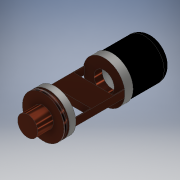
# Autodesk Inventor part: Part 3 of Focusrite Microphone
Saved by Autodesk Inventor 2018 (Build 220112000, 112)
## iProperties
Created: 2017-11-13
Part Number: Part 3 of Focusrite Microphone
Material: Generic
Document SubType Name: Modeling
Designer: Justin
Density: 1 g/cm^3
Appearance: Default
Author: Justin
Autodesk Inventor part; units mm, degrees
ref_plane "YZ Plane" through (0, 0, 0) normal (1, 0, 0) x (0, 1, 0)
ref_plane "XZ Plane" through (0, 0, 0) normal (0, 1, 0) x (-1, 0, 0)
ref_plane "XY Plane" through (0, 0, 0) normal (0, 0, 1) x (1, 0, 0)
sketch "Sketch1" plane through (0, 0, 0) normal (0, 0, 1) x (1, 0, 0)
  line L0 (0, 0) -> (12.3503, 0)
  line L1 (12.3503, 0) -> (12.3503, 19)
  line L2 (12.3503, 19) -> (0, 19)
  line L3 (0, 19) -> (0, 0)
  line L4 (0, 19) -> (25.485, 19)
  line L5 (25.485, 19) -> (25.485, 22.5)
  line L6 (25.485, 22.5) -> (0, 22.5)
  line L7 (0, 22.5) -> (0, 19)
  line L8 (23.226, 22.5) -> (23.226, 25.5)
  line L9 (23.226, 25.5) -> (0, 25.5)
  line L10 (0, 25.5) -> (0, 22.5)
  line L11 (23.226, 25.5) -> (25.485, 25.5)
  line L12 (25.485, 25.5) -> (25.485, 33.5)
  line L13 (25.485, 33.5) -> (20.485, 33.5)
  line L14 (20.485, 33.5) -> (20.485, 22.5)
  dimension "d0" = 19
  dimension "d1" = 25.485
  dimension "d2" = 3.5
  dimension "d3" = 90
  dimension "d4" = 3
  dimension "d5" = 8
  dimension "d6" = 5
  constraints: 30 end point, 11 perpendicular, 5 point on line, 1 horizontal, 1 parallel
  measures "d0" distance of L0.end L1.end
  measures "d1" distance of L2.end L4.end
  measures "d2" distance of L4.end L5.end
  measures "d3" angle of L5 L4
  measures "d4" distance of L8.start L8.end
  measures "d5" distance of L11.end L12.end
  measures "d6" distance of L12.end L13.end
revolve "Revolution1" add sketch "Sketch1" angle 360 about axis through (0, 19, 0) along (0, -1, 0)
sketch "Sketch2" plane through (0, 33.5, 0) normal (0, 1, 0) x (1, 0, 0)
  line L0 (25.0712, -4.4185) -> (24.0712, -4.4185)
  line L1 (24.0712, -4.4185) -> (24.0712, 4.5815)
  line L2 (24.0712, 4.5815) -> (25.0712, 4.5815)
  line L3 (25.0712, 4.5815) -> (25.0712, -4.4185)
  line L4 (-23.9768, -4.4185) -> (-24.9768, -4.4185)
  line L5 (-24.9768, -4.4185) -> (-24.9768, 4.5815)
  line L6 (-24.9768, 4.5815) -> (-23.9768, 4.5815)
  line L7 (-23.9768, 4.5815) -> (-23.9768, -4.4185)
  point P0 (0, 0)
  dimension "d8" = 1
  dimension "d9" = 9
  dimension "d10" = 1
  dimension "d11" = 9
  constraints: 16 end point, 4 parallel, 2 horizontal, 2 perpendicular, 1 point on line
  measures "d8" distance of L1.end L2.end
  measures "d9" distance of L0.end L1.end
  measures "d10" distance of L5.end L6.end
  measures "d11" distance of L4.end L5.end
extrude "Extrusion1" add sketch "Sketch2" along normal blind 60
sketch "Sketch3" plane through (0, 93.5, 0) normal (0, 1, 0) x (1, 0, 0)
  circle A0 centre (0, 0) radius 12.3503 projected
  circle A1 centre (0, 0) radius 25.485
  constraints: 1 centre point, 1 coincident
extrude "Extrusion2" add sketch "Sketch3" along normal blind 10
sketch "Sketch4" plane through (0, 103.5, 0) normal (0, 1, 0) x (1, 0, 0)
  point P0 (0, 0)
sketch "Sketch5" plane through (0, 103.5, 0) normal (0, 1, 0) x (1, 0, 0)
  circle A0 centre (0, 0) radius 24.5
  dimension "d16" = 49
  constraints: 1 centre point, 1 coincident
  measures "d16" diameter of A0
extrude "Extrusion3" add sketch "Sketch5" along normal blind 49
fillet "Fillet1" radius 10 1 edges at (-24.5, 152.5, 0)
sketch "Sketch6" plane through (-23.9768, 33.5, 4.4185) normal (1, 0, 0) x (0, 0, -1)
  line L0 (0, 0) -> (0, 60) projected
  line L1 (9, 0) -> (9, 60) projected
  line L2 (0, 19.4645) -> (9, 19.4645)
  line L3 (9, 19.4645) -> (9, 46.9149)
  line L4 (9, 46.9149) -> (0, 46.9149)
  line L5 (0, 46.9149) -> (0, 19.4645)
  point P0 (4.4185, -33.5)
  constraints: 8 end point, 2 parallel, 2 point on line, 1 horizontal, 1 perpendicular
extrude "Extrusion4" add sketch "Sketch6" along normal blind 49
thread "Thread1" size "M52x5" class "6g" standard "ANSI Metric M Profile" full length
body "Solid1"
